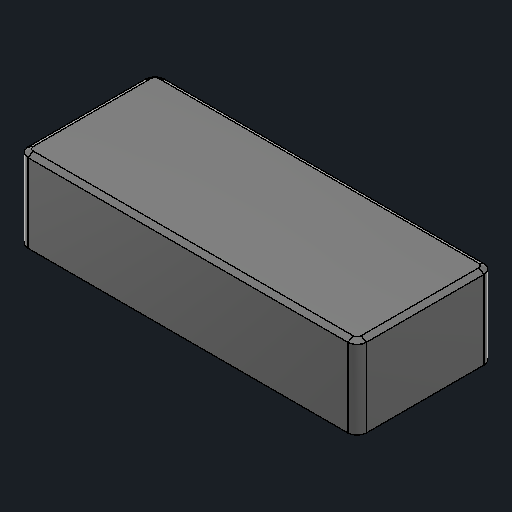
# Autodesk Inventor part: PS-24 PSU
Saved by Autodesk Inventor 2026.2 (Build 302298000, 298)
## iProperties
Created: 2026-08-15
Part Number: PS-24 PSU
Material: PC/ABS Plastic
Document SubType Name: Modeling
Designer: JoshuaEah
Density: 1.1 g/cm^3
Appearance: Smooth - Black
Author: JoshuaEah
Autodesk Inventor part; units mm, degrees
ref_plane "YZ Plane" through (0, 0, 0) normal (1, 0, 0) x (0, 1, 0)
ref_plane "XZ Plane" through (0, 0, 0) normal (0, 1, 0) x (-1, 0, 0)
ref_plane "XY Plane" through (0, 0, 0) normal (0, 0, 1) x (1, 0, 0)
sketch "Sketch1" plane through (0, 0, 0) normal (0, 1, 0) x (-1, 0, 0)
  line L0 (0, 0) -> (-128, 0)
  line L1 (-128, 0) -> (-128, -51.5)
  line L2 (-128, -51.5) -> (0, -51.5)
  line L3 (0, -51.5) -> (0, 0)
  dimension "d0" = 128
  dimension "d1" = 51.5
  constraints: 8 end point, 2 parallel, 1 coincident, 1 horizontal, 1 perpendicular
  measures "d0" distance of L1.end L2.end
  measures "d1" distance of L0.end L1.end
extrude "Extrusion1" add sketch "Sketch1" along normal blind 32
fillet "Fillet1" radius 3.5 4 edges at (128, 16, 0) (128, 16, -51.5) (0, 16, 0) (0, 16, -51.5)
chamfer "Chamfer1" distance 2 angle 30 4 edges at (64, 32, 0) (0, 32, -25.75) (64, 32, -51.5) (128, 32, -25.75) measured on face at (43.8333, 32, -34.3333)
chamfer "Chamfer2" distance 2 angle 30 4 edges at (64, 0, 0) (128, 0, -25.75) (64, 0, -51.5) (0, 0, -25.75) measured on face at (43.8333, 0, -34.3333)
body "Solid1"
